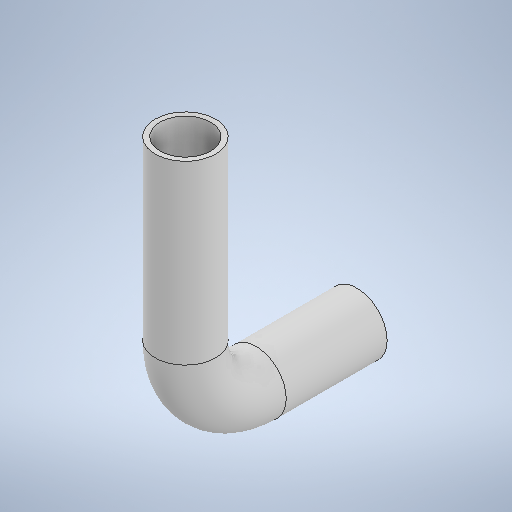
# Autodesk Inventor part: 24
Saved by Autodesk Inventor 2025.1 (Build 291241000, 241)
## iProperties
Created: 2024-09-13
Part Number: 24
Material: Generisch
Document SubType Name: Modeling
Designer: ffogue
Density: 1 g/cm^3
Appearance: Vorgabe
Author: ffogue
Autodesk Inventor part; units mm, degrees
ref_plane "YZ Plane" through (0, 0, 0) normal (1, 0, 0) x (0, 1, 0)
ref_plane "XZ Plane" through (0, 0, 0) normal (0, 1, 0) x (-1, 0, 0)
ref_plane "XY Plane" through (0, 0, 0) normal (0, 0, 1) x (1, 0, 0)
sketch "Sketch1" plane through (0, 0, 0) normal (0, 1, 0) x (-1, 0, 0)
  circle A0 centre (0, 0) radius 3
  circle A1 centre (0, 0) radius 2.5
  dimension "d0" = 6
  dimension "d4" = 5
  constraints: 2 centre point, 2 coincident
  measures "d0" diameter of A0
  measures "d4" diameter of A1
sketch "Sketch2" plane through (0, 0, 0) normal (1, 0, 0) x (0, 1, 0)
  line L0 (0, 0) -> (-10, 0)
  arc A0 (-17, 7) -> (-10, 0) centre (-10, 7) ccw
  line L1 (-17, 7) -> (-17, 24.5)
  line L2 (0, -3) -> (0, 3) projected
  dimension "d1" = 24.5
  dimension "d2" = 7
  dimension "d3" = 17
  constraints: 4 end point, 2 point on circle, 2 tangent, 1 centre point, 1 horizontal, 1 midpoint, 1 perpendicular
  measures "d1" vertical distance of L1.end point (0, 0)
  measures "d2" radius of A0
  measures "d3" horizontal distance of L1.end L2.end
sweep "Sweep1" add profiles "Sketch1" path "Sketch2" path curves L0 A0 L1
body "Solid1"
